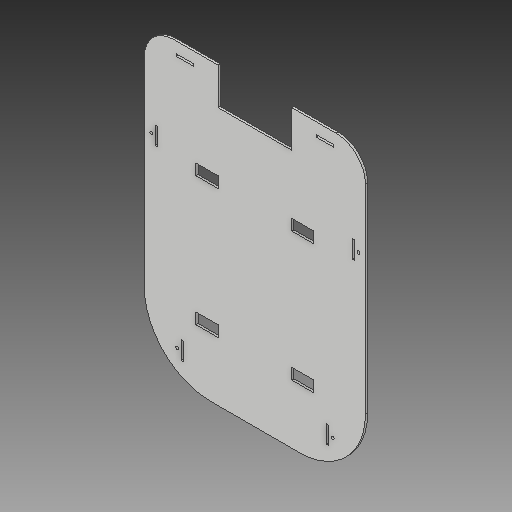
# Autodesk Inventor part: Top plate
Saved by Autodesk Inventor 2018 (Build 220112000, 112)
## iProperties
Created: 2018-05-03
Part Number: Top plate
Material: Generic
Document SubType Name: Modeling
Designer: Ajith Thomas
Density: 1 g/cm^3
Appearance: Default
Author: Ajith Thomas
Autodesk Inventor part; units mm, degrees
ref_plane "YZ Plane" through (0, 0, 0) normal (1, 0, 0) x (0, 1, 0)
ref_plane "XZ Plane" through (0, 0, 0) normal (0, 1, 0) x (-1, 0, 0)
ref_plane "XY Plane" through (0, 0, 0) normal (0, 0, 1) x (1, 0, 0)
sketch "Sketch1" plane through (0, 0, 0) normal (0, 0, 1) x (1, 0, 0)
  line L0 (0, 0) -> (0, 24) projected
  line L1 (3, 0) -> (0, 0) projected
  line L2 (3, 24) -> (3, 0) projected
  line L3 (0, 24) -> (3, 24) projected
  circle A0 centre (8.5, 12) radius 2 projected
  line L4 (-35, -235) -> (-35, -211) projected
  line L5 (-32, -235) -> (-35, -235) projected
  line L6 (-32, -211) -> (-32, -235) projected
  line L7 (-35, -211) -> (-32, -211) projected
  circle A1 centre (-26.5, -223) radius 2 projected
  line L8 (-232, -235) -> (-232, -211) projected
  line L9 (-229, -235) -> (-232, -235) projected
  line L10 (-229, -211) -> (-229, -235) projected
  line L11 (-232, -211) -> (-229, -211) projected
  circle A2 centre (-237.5, -223) radius 2 projected
  line L12 (-267, 0) -> (-267, 24) projected
  line L13 (-264, 0) -> (-267, 0) projected
  line L14 (-264, 24) -> (-264, 0) projected
  line L15 (-267, 24) -> (-264, 24) projected
  circle A3 centre (-272.5, 12) radius 2 projected
  line L16 (-215, 119) -> (-239, 119) projected
  line L17 (-215, 122) -> (-215, 119) projected
  line L18 (-239, 122) -> (-215, 122) projected
  line L19 (-239, 119) -> (-239, 122) projected
  line L20 (-25, 119) -> (-49, 119) projected
  line L21 (-25, 122) -> (-25, 119) projected
  line L22 (-49, 122) -> (-25, 122) projected
  line L23 (-49, 119) -> (-49, 122) projected
  line L24 (-22, 137) -> (-242, 137) projected
  arc A4 (18, 97) -> (-22, 137) centre (-22, 97) ccw projected
  line L25 (18, -173) -> (18, 97) projected
  arc A5 (-72, -263) -> (18, -173) centre (-72, -173) ccw projected
  line L26 (-192, -263) -> (-72, -263) projected
  arc A6 (-282, -173) -> (-192, -263) centre (-192, -173) ccw projected
  line L27 (-282, 97) -> (-282, -173) projected
  arc A7 (-242, 137) -> (-282, 97) centre (-242, 97) ccw projected
  line L28 (-132, 137) -> (-132, -263) construction
  line L29 (-132, 87) -> (-82, 87)
  line L30 (-82, 87) -> (-82, 137)
  line L31 (-132, 87) -> (-182, 87)
  line L32 (-182, 87) -> (-182, 137)
  line L33 (-82, 137) -> (-182, 137)
  dimension "d0" = 50
  dimension "d1" = 50
  constraints: 12 end point, 2 midpoint, 2 perpendicular, 2 point on line, 2 symmetric about line, 1 horizontal
  measures "d0" distance between parallel lines of L24 L29
  measures "d1" distance between parallel lines of L28 L30
extrude "Extrusion1" add sketch "Sketch1" against normal blind 3 contours A4 L25 A5 L26 A6 L27 A7 L24 L32 L31 L29 L30
sketch "Sketch2" plane through (0, 0, 0) normal (0, 0, 1) x (1, 0, 0)
  line L0 (-82, 87) -> (-182, 87) projected
  line L1 (-192, -263) -> (-72, -263) projected
  line L2 (18, -173) -> (18, 97) projected
  line L3 (-282, 97) -> (-282, -173) projected
  line L4 (-132, 87) -> (-132, -263) construction
  line L5 (-52, 7) -> (-82, 7)
  line L6 (-82, 7) -> (-82, -8)
  line L7 (-82, -8) -> (-52, -8)
  line L8 (-52, -8) -> (-52, 7)
  line L9 (-212, 7) -> (-182, 7)
  line L10 (-182, 7) -> (-182, -8)
  line L11 (-182, -8) -> (-212, -8)
  line L12 (-212, -8) -> (-212, 7)
  line L13 (-132, -88) -> (18, -88) construction
  line L14 (-52, -183) -> (-82, -183)
  line L15 (-82, -183) -> (-82, -168)
  line L16 (-82, -168) -> (-52, -168)
  line L17 (-52, -168) -> (-52, -183)
  line L18 (-182, -168) -> (-212, -168)
  line L19 (-182, -183) -> (-182, -168)
  line L20 (-212, -183) -> (-182, -183)
  line L21 (-212, -168) -> (-212, -183)
  point P0 (0, 0)
  dimension "d4" = 30
  dimension "d5" = 15
  dimension "d6" = 50
  dimension "d7" = 80
  constraints: 36 end point, 12 symmetric about line, 3 midpoint, 2 horizontal, 2 parallel, 1 perpendicular, 1 point on line
  measures "d4" distance of L7.end L6.end
  measures "d5" distance of L6.end L5.end
  measures "d6" distance between parallel lines of L4 L6
  measures "d7" distance between parallel lines of L0 L5
extrude "Extrusion2" cut sketch "Sketch2" against normal blind 3
body "Solid1"
